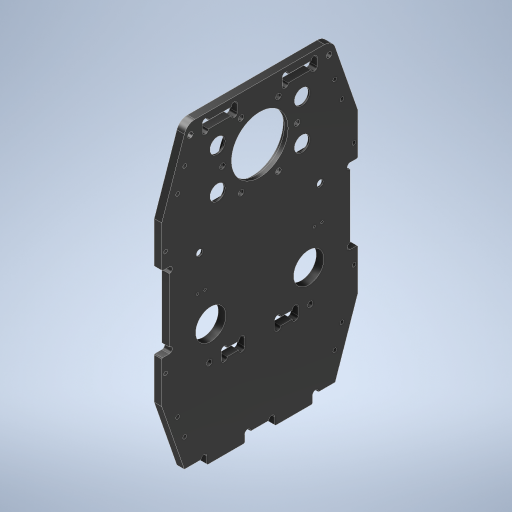
# Autodesk Inventor part: TorsoSideFrame
Saved by Autodesk Inventor 2024.2 (Build 282272000, 272)
## iProperties
Created: 2024-01-27
Part Number: TorsoSideFrame
Material: Aluminum 7075
Document SubType Name: Modeling
Designer: Masato Kubotera
Density: 2.81 g/cm^3
Appearance: Glossy - Black
Mass: 135.554 g
Surface Area: 564.093 cm^2
Volume: 48.24 cm^3
Vendor: meviy
Author: Masato Kubotera
Autodesk Inventor part; units mm, degrees
ref_plane "YZ Plane" through (0, 0, 0) normal (1, 0, 0) x (0, 1, 0)
ref_plane "XZ Plane" through (0, 0, 0) normal (0, 1, 0) x (-1, 0, 0)
ref_plane "XY Plane" through (0, 0, 0) normal (0, 0, 1) x (1, 0, 0)
sketch "Sketch1" plane through (0, 0, 0) normal (0, 1, 0) x (-1, 0, 0)
  circle A0 centre (0, 0) radius 18.75
  line L0 (0, 0) -> (0, -161.5)
  circle A1 centre (0, 0) radius 29 construction
  line L1 (0, 0) -> (0, 36)
  line L2 (0, 36) -> (-48.2759, 36)
  line L3 (-65, -12.5) -> (-65, -118)
  line L4 (-50, -161.5) -> (-35, -161.5)
  line L5 (-35, -161.5) -> (-35, -166.5)
  line L6 (-35, -166.5) -> (-10, -166.5)
  line L7 (-10, -166.5) -> (-10, -161.5)
  line L8 (-10, -161.5) -> (0, -161.5)
  line L9 (-60, -40.225) -> (-65, -40.225)
  line L10 (-44, -161.5) -> (-44, -155.5) construction
  line L11 (-22.5, -166.5) -> (-22.5, -161.5) construction
  arc A2 (-6, -161.5) -> (-10, -161.5) centre (-8, -161.5) ccw
  arc A3 (-35, -161.5) -> (-39, -161.5) centre (-37, -161.5) ccw
  line L12 (-65, -12.5) -> (-60, -12.5) construction
  line L13 (-60, -12.5) -> (-60, -106) construction
  line L14 (-62.5, -12.5) -> (-62.5, -106) construction
  line L15 (-65, -40.25) -> (-60, -40.25) construction
  arc A4 (-60, -44.225) -> (-60, -40.225) centre (-60, -42.225) ccw
  line L16 (-60, -111) -> (0, -111) construction
  line L17 (-60, -106) -> (0, -106) construction
  line L18 (-60, -108.5) -> (-17.75, -108.5) construction
  line L19 (-9.95, -111.05) -> (-25.55, -111.05)
  line L20 (-25.55, -111.05) -> (-25.55, -105.95)
  line L21 (-25.55, -105.95) -> (-9.95, -105.95)
  line L22 (-9.95, -105.95) -> (-9.95, -111.05)
  line L23 (-9.95, -111.05) -> (-25.55, -105.95) construction
  line L24 (-25.55, -111.05) -> (-9.95, -105.95) construction
  line L25 (-25.5, -106) -> (-25.5, -111) construction
  arc A5 (-21.55, -105.95) -> (-25.55, -105.95) centre (-23.55, -105.95) ccw
  arc A6 (-25.55, -111.05) -> (-21.55, -111.05) centre (-23.55, -111.05) ccw
  line L26 (-22.5, -76.875) -> (-42.5, -76.875) construction
  line L27 (-42.5, -76.875) -> (-42.5, -96.875) construction
  line L28 (-42.5, -96.875) -> (-22.5, -96.875) construction
  line L29 (-22.5, -96.875) -> (-22.5, -76.875) construction
  line L30 (-22.5, -76.875) -> (-42.5, -96.875) construction
  line L31 (-42.5, -76.875) -> (-22.5, -96.875) construction
  line L32 (-45, -74.375) -> (-20, -74.375) construction
  line L33 (-20, -74.375) -> (-20, -99.375) construction
  line L34 (-20, -99.375) -> (-45, -99.375) construction
  line L35 (-45, -99.375) -> (-45, -74.375) construction
  line L36 (-45, -74.375) -> (-20, -99.375) construction
  line L37 (-20, -74.375) -> (-45, -99.375) construction
  line L38 (-50, 31) -> (0, 31) construction
  line L39 (-38.05, 31.05) -> (-14.95, 31.05)
  line L40 (-14.95, 31.05) -> (-14.95, 25.95)
  line L41 (-14.95, 25.95) -> (-38.05, 25.95)
  line L42 (-38.05, 25.95) -> (-38.05, 31.05)
  line L43 (-38.05, 31.05) -> (-14.95, 25.95) construction
  line L44 (-14.95, 31.05) -> (-38.05, 25.95) construction
  line L45 (-38.05, 28.5) -> (-14.95, 28.5) construction
  line L46 (-38, 31) -> (-38, 26) construction
  line L47 (-26.5, 31.05) -> (-26.5, 25.95) construction
  line L48 (-15, 31) -> (-15, 26) construction
  arc A7 (-34.05, 31.05) -> (-38.05, 31.05) centre (-36.05, 31.05) ccw
  arc A8 (-38.05, 25.95) -> (-34.05, 25.95) centre (-36.05, 25.95) ccw
  arc A9 (-14.95, 31.05) -> (-18.95, 31.05) centre (-16.95, 31.05) ccw
  arc A10 (-18.95, 25.95) -> (-14.95, 25.95) centre (-16.95, 25.95) ccw
  line L49 (-46.4119, -155.5) -> (-3.5, -155.5)
  arc A11 (-48.3027, -154.152) -> (-46.4119, -155.5) centre (-46.4119, -153.5) ccw
  arc A12 (-3.5, -155.5) -> (-1.5, -153.5) centre (-3.5, -153.5) ccw
  circle A13 centre (-41.25, -65.25) radius 2 construction
  line L50 (-3.5, -62.75) -> (-54, -62.75)
  line L51 (0, 0) -> (-29, 0) construction
  line L52 (-30.7958, -111) -> (-29.7506, -111)
  arc A14 (-27.8427, -112.4) -> (-20.2699, -114.1308) centre (-23.55, -111.05) ccw
  line L53 (-1.5, -153.5) -> (-1.5, -113)
  arc A15 (-1.5, -113) -> (-3.5, -111) centre (-3.5, -113) ccw
  arc A16 (-27.8427, -112.4) -> (-29.7506, -111) centre (-29.7506, -113) ccw
  circle A17 centre (-33.5, -108.5) radius 1.75 construction
  arc A18 (-18.8121, -113.5) -> (-20.2699, -114.1308) centre (-18.8121, -115.5) ccw
  line L54 (-17.75, -105.95) -> (-17.75, -111.05) construction
  arc A19 (-20.2699, -102.8692) -> (-27.8427, -104.6) centre (-23.55, -105.95) ccw
  arc A20 (-29.7506, -106) -> (-27.8427, -104.6) centre (-29.7506, -104) ccw
  arc A21 (-20.2699, -102.8692) -> (-18.8121, -103.5) centre (-18.8121, -101.5) ccw
  line L55 (-10, -106) -> (-10, -111) construction
  arc A22 (-9.95, -105.95) -> (-13.95, -105.95) centre (-11.95, -105.95) ccw
  arc A23 (-13.95, -111.05) -> (-9.95, -111.05) centre (-11.95, -111.05) ccw
  arc A24 (-15.2301, -114.1308) -> (-7.6573, -112.4) centre (-11.95, -111.05) ccw
  arc A25 (-5.7494, -111) -> (-7.6573, -112.4) centre (-5.7494, -113) ccw
  arc A26 (-15.2301, -114.1308) -> (-16.6879, -113.5) centre (-16.6879, -115.5) ccw
  arc A27 (-7.6573, -104.6) -> (-5.7494, -106) centre (-5.7494, -104) ccw
  arc A28 (-7.6573, -104.6) -> (-15.2301, -102.8692) centre (-11.95, -105.95) ccw
  arc A29 (-16.6879, -103.5) -> (-15.2301, -102.8692) centre (-16.6879, -101.5) ccw
  line L56 (-18.8121, -103.5) -> (-16.6879, -103.5)
  line L57 (-18.8121, -113.5) -> (-16.6879, -113.5)
  line L58 (-5.7494, -111) -> (-3.5, -111)
  arc A30 (-3.5, -106) -> (-1.5, -104) centre (-3.5, -104) ccw
  line L59 (-5.7494, -106) -> (-3.5, -106)
  line L60 (-41.25, -65.25) -> (-36.25, -65.25) construction
  line L61 (-60, -44.225) -> (-60, -86.275)
  line L62 (-60, -65.25) -> (-65, -65.25) construction
  line L63 (-60, -90.275) -> (-65, -90.275)
  line L64 (-65, -90.25) -> (-60, -90.25) construction
  arc A31 (-60, -90.275) -> (-60, -86.275) centre (-60, -88.275) ccw
  line L65 (-60, -106) -> (-65, -106) construction
  line L66 (-1.5, -24.2487) -> (-1.5, -60.75)
  line L67 (-54, -67.75) -> (-3.5, -67.75)
  line L68 (-1.5, -69.75) -> (-1.5, -104)
  line L69 (-56, -60.75) -> (-56, -47.5165)
  circle A32 centre (-32.5, -86.875) radius 10
  circle A33 centre (-32.5, -86.875) radius 11
  arc A34 (-15.79, 16.0289) -> (-21.7764, 5.6601) centre (0, 0) ccw
  arc A35 (-21.7764, -5.6601) -> (-15.79, -16.0289) centre (0, 0) ccw
  arc A36 (-5.9864, -21.689) -> (-3.2143, -22.2692) centre (0, 0) ccw
  arc A37 (-24.0442, 4.191) -> (-24.0442, -4.191) centre (-24.75, 0) ccw
  line L70 (-48.2759, 36) -> (-65, -12.5)
  arc A38 (-42.9869, 36) -> (-50, 31) centre (-42.9869, 28.5817) ccw
  ellipse E0 centre (-84.0749, 16.6972) end of major axis (-93.0397, -9.3006) minor radius 20 construction
  line L71 (-75.1102, 42.6949) -> (-76.7401, 37.9681) construction
  line L72 (-105, 43.5) -> (-105, 11.4504) construction
  ellipse E1 centre (-84.0749, 16.6972) end of major axis (-76.7401, 37.9681) minor radius 15 construction
  line L73 (-75.1102, 42.6949) -> (-93.0397, -9.3006) construction
  line L74 (-84.0749, 16.6972) -> (-58.029, 7.7158) construction
  line L75 (-63.4041, 25.9649) -> (-39.2683, 17.6422) construction
  line L76 (-39.2683, 17.6422) -> (-49.374, -11.6643) construction
  line L77 (-49.374, -11.6643) -> (-73.5098, -3.3416) construction
  line L78 (-79.9787, 43.5) -> (-105, 43.5) construction
  line L79 (-47.0676, 20.3317) -> (-57.1733, -8.9749) construction
  circle A39 centre (-49.757, 12.5323) radius 6.25 construction
  circle A40 centre (-54.4839, -1.1756) radius 6.25 construction
  line L80 (-1, 13.5) -> (-28, 13.5) construction
  line L81 (-28, 13.5) -> (-28, -13.5) construction
  line L82 (-28, -13.5) -> (-1, -13.5) construction
  line L83 (-1, -13.5) -> (-1, 13.5) construction
  line L84 (-1, 13.5) -> (-28, -13.5) construction
  line L85 (-28, 13.5) -> (-1, -13.5) construction
  line L86 (0, -65.25) -> (-64.9996, -65.25) construction
  line L87 (-50, -161.5) -> (-65, -118)
  line L88 (-18.3182, 21.5) -> (-45.3395, 21.5)
  arc A41 (-16.4164, 20.1189) -> (-15.6516, 18.7274) centre (-12.375, 21.4341) ccw
  arc A42 (-55.5, -46.1936) -> (-58.5, -36.4155) centre (-60, -42.225) ccw
  arc A43 (-48.7278, 6.3677) -> (-46.4104, 17.8109) centre (-49.757, 12.5323) ccw
  arc A44 (-48.7278, 6.3677) -> (-49.8737, 3.0445) centre (-48.3985, 4.395) ccw
  arc A45 (-56.6994, -7.0197) -> (-49.8737, 3.0445) centre (-54.4839, -1.1756) ccw
  line L89 (-38, 26) -> (-15, 26) construction
  line L90 (-59.2992, -8.2378) -> (-59.8907, -9.9535)
  arc A46 (-47.8996, -149) -> (-48.7278, -136.8677) centre (-49.757, -143.0323) ccw
  arc A47 (-49.8737, -133.5445) -> (-48.7278, -136.8677) centre (-48.3985, -134.895) ccw
  arc A48 (-49.8737, -133.5445) -> (-56.6994, -123.4803) centre (-54.4839, -129.3244) ccw
  line L91 (-48.3027, -154.152) -> (-49.1959, -151.5616)
  line L92 (-59.2992, -122.2622) -> (-59.8907, -120.5465)
  line L93 (-60, -119.8946) -> (-60, -113)
  circle A49 centre (-41.25, -65.25) radius 1 construction
  line L94 (-45, -86.875) -> (-20, -86.875) construction
  arc A50 (-45.3395, 21.5) -> (-46.4104, 17.8109) centre (-45.3395, 19.5) ccw
  arc A51 (-56.6994, -7.0197) -> (-59.2992, -8.2378) centre (-57.4084, -8.8898) ccw
  arc A52 (-16.4164, 20.1189) -> (-18.3182, 21.5) centre (-18.3182, 19.5) ccw
  arc A53 (-15.79, 16.0289) -> (-15.6516, 18.7274) centre (-17.1936, 17.4537) ccw
  arc A54 (-24.0442, 4.191) -> (-21.7764, 5.6601) centre (-23.7121, 6.1632) ccw
  arc A55 (-21.7764, -5.6601) -> (-24.0442, -4.191) centre (-23.7121, -6.1632) ccw
  arc A56 (-15.6516, -18.7274) -> (-15.79, -16.0289) centre (-17.1936, -17.4537) ccw
  arc A57 (-5.9864, -21.689) -> (-8.3926, -22.9184) centre (-6.5186, -23.6169) ccw
  arc A58 (-60, -34.479) -> (-58.5, -36.4155) centre (-58, -34.479) ccw
  line L95 (-40, -42.225) -> (-60, -42.225) construction
  circle A59 centre (-33.5, -108.5) radius 3.25 construction
  arc A60 (-35.174, -111.2857) -> (-31.826, -111.2857) centre (-33.5, -108.5) ccw
  line L96 (-36.2042, -111) -> (-58, -111)
  arc A61 (-31.826, -105.7143) -> (-35.174, -105.7143) centre (-33.5, -108.5) ccw
  line L97 (-36.2042, -106) -> (-58, -106)
  line L98 (-30.7958, -106) -> (-29.7506, -106)
  arc A62 (-58.5, -94.0845) -> (-55.5, -84.3064) centre (-60, -88.275) ccw
  arc A63 (-58.5, -94.0845) -> (-60, -96.021) centre (-58, -96.021) ccw
  line L99 (-56, -69.75) -> (-56, -82.9835)
  line L100 (-60, -96.021) -> (-60, -104)
  arc A64 (-36.2042, -106) -> (-35.174, -105.7143) centre (-36.2042, -104) ccw
  arc A65 (-35.174, -111.2857) -> (-36.2042, -111) centre (-36.2042, -113) ccw
  arc A66 (-60, -104) -> (-58, -106) centre (-58, -104) ccw
  arc A67 (-58, -111) -> (-60, -113) centre (-58, -113) ccw
  circle A68 centre (-36.25, -65.25) radius 2 construction
  arc A69 (-31.826, -105.7143) -> (-30.7958, -106) centre (-30.7958, -104) ccw
  arc A70 (-30.7958, -111) -> (-31.826, -111.2857) centre (-30.7958, -113) ccw
  arc A71 (-47.8996, -149) -> (-49.1959, -151.5616) centre (-47.3052, -150.9096) ccw
  arc A72 (-59.2992, -122.2622) -> (-56.6994, -123.4803) centre (-57.4084, -121.6102) ccw
  arc A73 (-60, -119.8946) -> (-59.8907, -120.5465) centre (-58, -119.8946) ccw
  arc A74 (-60, -119.8946) -> (-59.8907, -120.5465) centre (-58, -119.8946) ccw
  arc A75 (-56, -82.9835) -> (-55.5, -84.3064) centre (-54, -82.9835) ccw
  arc A76 (-54, -67.75) -> (-56, -69.75) centre (-54, -69.75) ccw
  arc A77 (-56, -60.75) -> (-54, -62.75) centre (-54, -60.75) ccw
  arc A78 (-55.5, -46.1936) -> (-56, -47.5165) centre (-54, -47.5165) ccw
  arc A79 (-1.5, -69.75) -> (-3.5, -67.75) centre (-3.5, -69.75) ccw
  arc A80 (-3.5, -62.75) -> (-1.5, -60.75) centre (-3.5, -60.75) ccw
  line L101 (-18.3182, -21.5) -> (-58, -21.5)
  arc A81 (-18.3182, -21.5) -> (-16.4164, -20.1189) centre (-18.3182, -19.5) ccw
  arc A82 (-15.6516, -18.7274) -> (-16.4164, -20.1189) centre (-12.375, -21.4341) ccw
  arc A83 (-14.5, -25.1147) -> (-8.3926, -22.9184) centre (-12.375, -21.4341) ccw
  line L102 (-16.0857, -24.5) -> (-58, -24.5)
  arc A84 (-1.5, -24.2487) -> (-3.2143, -22.2692) centre (-3.5, -24.2487) ccw
  line L103 (-60, -10.6054) -> (-60, -19.5)
  line L104 (-60, -26.5) -> (-60, -34.479)
  arc A85 (-59.8907, -9.9535) -> (-60, -10.6054) centre (-58, -10.6054) ccw
  arc A86 (-60, -19.5) -> (-58, -21.5) centre (-58, -19.5) ccw
  arc A87 (-58, -24.5) -> (-60, -26.5) centre (-58, -26.5) ccw
  arc A88 (-15.0479, -24.7903) -> (-14.5, -25.1147) centre (0, 0) ccw
  arc A89 (-15.0479, -24.7903) -> (-16.0857, -24.5) centre (-16.0857, -26.5) ccw
  point P0 (-16.05, -9.6933)
  point P1 (-12.375, -21.4341)
  point P2 (12.375, -21.4341)
  point P3 (24.75, 0)
  point P4 (12.375, 21.4341)
  point P5 (-26.5, 28.5)
  point P6 (0, -18.75)
  point P7 (0, 18.75)
  point P8 (0, -106.55)
  point P9 (-21.55, -111.05)
  point P10 (0, -101.45)
  point P11 (-18.95, 25.95)
  point P12 (-34.05, 25.95)
  point P13 (-60, -106)
  point P14 (-46, 28.5)
  point P15 (-35.05, 18.95)
  point P16 (-56, -62.75)
  point P17 (-1.5, -155.5)
  point P18 (-5, -161.5)
  point P19 (-28.0497, -111)
  point P20 (-28.0239, -110.5665)
  point P21 (-1.5, -62.75)
  point P22 (-7.4503, -111)
  point P23 (-13.95, -105.95)
  point P24 (-13.95, -111.05)
  point P25 (-65, -90.275)
  point P26 (-56, -67.75)
  point P27 (-1.5, -67.75)
  point P28 (-1.5, -22.4499)
  point P29 (-38, 28.5)
  point P30 (-14.5, 0)
  point P31 (-1, 0)
  point P32 (-50, -161.5)
  point P33 (-16.6245, 21.5)
  point P34 (-56, -46.6971)
  point P35 (-60, -36.225)
  point P36 (-49.9833, 18.7782)
  point P37 (-58.5118, -5.9545)
  point P38 (-60, -10.2703)
  point P39 (-62.5, -30.25)
  point P40 (-62.5, -100.25)
  point P41 (-49.9833, -149.2782)
  point P42 (-58.5118, -124.5455)
  point P43 (-60, -120.2297)
  point P44 (-37.0826, -67.75)
  point P45 (-27.9174, -67.75)
  point P46 (-32.5, -67.75)
  point P47 (-36.05, 23.95)
  point P48 (-31.4233, -111)
  point P49 (-31.4233, -106)
  point P50 (-56, -83.8029)
  point P51 (-40, -88.275)
  point P52 (-15.5161, -24.5)
  dimension "d0" = 37.5
  dimension "d198" = 20
  dimension "d202" = 15
  dimension "d219" = 12.5
  dimension "d1" = 161.5
  dimension "d2" = 58
  dimension "d16" = 360
  dimension "d18" = 49.5
  dimension "d20" = 20
  dimension "d21" = 5
  dimension "d23" = 6
  dimension "d24" = 0.025
  dimension "d26" = 5
  dimension "d27" = 21.25
  dimension "d31" = 5
  dimension "d32" = 50.5
  dimension "d34" = 0.05
  dimension "d35" = 2
  dimension "d36" = 0.05
  dimension "d37" = 8
  dimension "d38" = 20
  dimension "d39" = 20
  dimension "d40" = 25
  dimension "d41" = 25
  dimension "d52" = 0.05
  dimension "d53" = 0.05
  dimension "d105" = 4
  dimension "d108" = 8
  dimension "d136" = 3.5
  dimension "d142" = 3
  dimension "d156" = 2.5
  dimension "d157" = 2.5
  dimension "d158" = 15.5
  dimension "d160" = 50
  dimension "d162" = 5
  dimension "d167" = 20
  dimension "d169" = 65
  dimension "d171" = 20
  dimension "d180" = 1
  dimension "d181" = 22.5
  dimension "d182" = 5
  dimension "d183" = 10
  dimension "d184" = 197.5
  dimension "d186" = 30
  dimension "d187" = 100
  dimension "d188" = 12
  dimension "d189" = 19.026
  dimension "d201" = 5
  dimension "d205" = 55
  dimension "d220" = 2
  dimension "d221" = 2
  dimension "d222" = 2
  dimension "d223" = 210
  dimension "d224" = 7.5
  dimension "d225" = 27
  dimension "d226" = 27
  dimension "d229" = 25
  dimension "d230" = 9
  dimension "d235" = 2
  dimension "d243" = 4
  dimension "d244" = 4
  dimension "d246" = 1
  dimension "d248" = 70
  dimension "d249" = 2
  dimension "d250" = 105.5
  dimension "d253" = 130
  dimension "d254" = 2
  dimension "d255" = 1.5
  constraints: 210 end point, 176 point on circle, 88 centre point, 78 tangent, 69 symmetric about line, 65 point on line, 40 equal radius, 30 horizontal, 28 midpoint, 23 coincident, 19 vertical, 13 parallel, 10 collinear, 7 perpendicular, 73 other
  measures "d1" distance of L0.start L0.end
  measures "d2" diameter of A1
  measures "d18" distance of point (24.75, 0) point (-24.75, 0)
  measures "d20" diameter of L7 L0
  measures "d21" distance of L4.end L5.end
  measures "d23" distance of L10.start L10.end
  measures "d24" distance between parallel lines of L9 L15
  measures "d26" distance of point (-36.25, -65.25) point (-41.25, -65.25)
  measures "d27" distance from line of point (-41.25, -65.25) L14
  measures "d31" distance between parallel lines of L16 L17
  measures "d32" distance between parallel lines of L4 L16
  measures "d34" distance between parallel lines of L17 L21
  measures "d35" radius of A4
  measures "d36" distance between parallel lines of L20 L25
  measures "d37" distance from line of L25 point (-33.5, -108.5)
  measures "d38" distance of L28.end L27.end
  measures "d39" distance of L27.end L26.end
  measures "d40" distance of L33.end L34.end
  measures "d41" distance of L32.end L33.end
  measures "d52" distance between parallel lines of L42 L46
  measures "d53" distance between parallel lines of L39 L38
  measures "d105" diameter of A13
  measures "d108" distance from line of point (-46, 28.5) L46
  measures "d136" diameter of A17
  measures "d142" diameter of L53 L0
  measures "d156" distance between parallel lines of L57 L16
  measures "d157" radial gap between concentric circles of A14 A6
  measures "d158" distance between parallel lines of L55 L25
  measures "d160" distance between parallel lines of L64 L15
  measures "d162" distance of L65.start L65.end
  measures "d167" diameter of L55 L0
  measures "d169" diameter of point (-32.5, -86.875) L0
  measures "d171" diameter of A32
  measures "d180" radial gap between concentric circles of A33 A32
  measures "d181" radius of A34
  measures "d182" distance of L46.start L46.end
  measures "d183" distance from line of L46.end L2
  measures "d184" distance between parallel lines of L2 L4
  measures "d186" diameter of L48 L1
  measures "d187" diameter of L38.start L1
  measures "d188" distance from line of L38.start L46
  measures "d189" angle of L3 L70
  measures "d201" distance of L73.start L71.end
  measures "d205" distance of L73.start L73.end
  measures "d223" diameter of L72 L1
  measures "d224" distance between parallel lines of L78 L2
  measures "d225" distance of L82.end L81.end
  measures "d226" distance of L81.end L80.end
  measures "d229" distance between parallel lines of L7 L5
  measures "d230" distance between parallel lines of L5 L10
  measures "d235" radius of A44
  measures "d243" radial gap between concentric circles of A42 A4
  measures "d246" distance between parallel lines of L83 L0
  measures "d248" distance of point (-62.5, -100.25) point (-62.5, -30.25)
  measures "d249" radius of A15
  measures "d250" distance of L3.end L3.start
  measures "d253" diameter of L3 L0
  measures "d254" diameter of A49
  measures "d255" distance edge to line of A49 L67
extrude "Extrusion1" add sketch "Sketch1" along normal blind 5 contours A0 L0 L8 A2 L7 L6 L5 A3 L4 L87 L3 L63 A31 L61 A4 L9 L70 A38 L2 L1 | A11 L91 A71 A46 A47 A48 A72 L92 A73 L93 A67 L96 A65 A60 A70 L52 A16 A14 A18 L57 A26 A24 A25 L58 A15 L53 A12 L49 | L50 A77 L69 A78 A42 A58 L104 A87 L102 A89 A88 A83 A57 A36 A84 L66 A80 | A19 A20 L98 A69 A61 A64 L97 A66 L100 A63 A62 A75 L99 A76 L67 A79 L68 A30 L59 A27 A28 A29 L56 A21 | A33 | A34 A54 A37 A55 A35 A56 A82 A81 L101 A86 L103 A85 L90 A51 A45 A44 A43 A50 L88 A52 A41 A53
extrude "Extrusion3" cut sketch "Sketch1" along normal blind 4 contours A11 L91 A71 A46 A47 A48 A72 L92 A73 L93 A67 L96 A65 A60 A70 L52 A16 A14 A18 L57 A26 A24 A25 L58 A15 L53 A12 L49 | L50 A77 L69 A78 A42 A58 L104 A87 L102 A89 A88 A83 A57 A36 A84 L66 A80 | A19 A20 L98 A69 A61 A64 L97 A66 L100 A63 A62 A75 L99 A76 L67 A79 L68 A30 L59 A27 A28 A29 L56 A21 | A34 A54 A37 A55 A35 A56 A82 A81 L101 A86 L103 A85 L90 A51 A45 A44 A43 A50 L88 A52 A41 A53
hole "M2" at (41.25, 0, -65.25) at (36.25, 0, -65.25) direction (0, 1, 0) diameter 1.567 end through all thread size "M2x0.4" class "6H" standard "ANSI Metric M Profile"
hole "M3" at (-24.75, 0, 0) at (-12.375, 0, 21.4341) at (49.757, 0, 12.5323) at (54.4839, 0, -1.1756) at (54.4839, 0, -129.3244) at (49.757, 0, -143.0323) at (62.5, 0, -30.25) at (62.5, 0, -100.25) direction (0, 1, 0) diameter 2.459 end through all thread size "M3x0.5" class "6H" standard "ANSI Metric M Profile"
hole "Ph3.5" at (33.5, 0, -108.5) at (46, 0, 28.5) direction (0, 1, 0) diameter 3.5 end through all
hole "Phi3.5-6.1" at (24.75, 0, 0) at (12.375, 0, -21.4341) at (-12.375, 0, -21.4341) at (12.375, 0, 21.4341) direction (0, 1, 0) diameter 3.5 end through all counterbore diameter 6.1 counterbore depth 3.5
hole "Phi41-H7" at (0, 0, 0) direction (0, 1, 0) diameter 41 depth 2.5
chamfer "C0.5" distance 0.5 angle 45 4 edges at (65, 2.5, -40.225) (35, 2.5, -166.5) (10, 2.5, -166.5) (65, 2.5, -90.275)
mirror "Mirror1" about plane through (0, 0, 0) normal (1, 0, 0)
hole "Phi10.0" at (28, 0, 13.5) at (28, 0, -13.5) direction (0, 1, 0) diameter 10 end through all
hole "Phi4.0" at (40, 0, -42.225) direction (0, 1, 0) diameter 4 end through all
sketch "Sketch3" plane through (6, 0, -161.5) normal (0, 0, -1) x (-1, 0, 0)
  line L0 (6, 0) -> (6, 5)
  line L1 (0, 5) -> (12, 5) projected
  line L2 (-38, 0) -> (-38, 5)
  line L3 (-44, 5) -> (-33, 5) projected
  point P0 (6, 2.5)
  point P1 (6, 2.5)
  point P2 (-38, 2.5)
  constraints: 4 end point, 3 midpoint, 1 coincident, 1 point on line, 1 vertical
hole "Bottom-M3" at (44, 2.5, -161.5) at (0, 2.5, -161.5) direction (0, 0, 1) diameter 2.459 depth 6 thread size "M3x0.5" class "6H" standard "ANSI Metric M Profile"
mirror "Mirror2" about plane through (0, 0, 0) normal (1, 0, 0) of "Phi10.0", "Phi4.0", "Bottom-M3"
body "Solid1"
